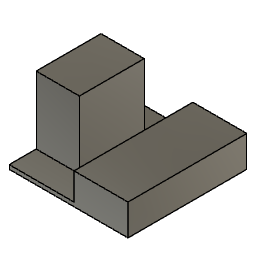
MotorDriver v2 (Autodesk Fusion 360 design; units mm, degrees)
Autodesk Fusion 360 part; units mm, degrees
sketch "Esquisse1" plane through (0, 0, 0) normal (0, 0, 1) x (1, 0, 0)
  line L0 (0, 0) -> (4.4, 0)
  line L1 (4.4, 0) -> (4.4, 4.4)
  line L2 (4.4, 4.4) -> (0, 4.4)
  line L3 (0, 4.4) -> (0, 0)
  dimension "d1" = 4.4
  dimension "d2" = 4.4
  constraint horizontal L0
  constraint vertical L1
  constraint horizontal L2
  constraint vertical L3
  constraint coincident L0.start L3.end
  measures "d1" distance of L0.start L0.end
  measures "d2" distance of L0.start L2.end
extrude "Extrusion1" add sketch "Esquisse1" along normal blind 0.15
sketch "Esquisse2" plane through (0, 0, 0.15) normal (0, 0, 1) x (-1, 0, 0)
  line L0 (0, -4.4) -> (0, 0)
  line L1 (0, 0) -> (-4.4, 0)
  line L2 (-4.4, 0) -> (-4.4, -4.4)
  line L3 (-4.4, -4.4) -> (0, -4.4)
  line L4 (-4.4, 0) -> (-2.4, 0)
  line L5 (-2.4, 0) -> (-2.4, -4.4)
  line L6 (-2.4, -4.4) -> (-4.4, -4.4)
  line L7 (-4.4, -4.4) -> (-4.4, 0)
  dimension "d5" = 2
  constraint horizontal L4
  constraint vertical L5
  constraint horizontal L6
  constraint vertical L7
  constraint coincident L3 L5.end
  constraint coincident L1.end L2.start
  measures "d5" distance of L1.end L4.end
extrude "Extrusion2" add sketch "Esquisse2" along normal blind 1 contours L1 L2 L3 L4 L5 L6 L7
sketch "Esquisse3" plane through (0, 0, 0.15) normal (0, 0, 1) x (-1, 0, 0)
  line L0 (-2.4, 0) -> (-2.4, -4.4)
  line L1 (-2.4, -4.4) -> (0, -4.4)
  line L2 (0, -4.4) -> (0, 0)
  line L3 (0, 0) -> (-2.4, 0)
  line L4 (0, -3.4) -> (-1.6, -3.4)
  line L5 (-1.6, -3.4) -> (-1.6, -1)
  line L6 (-1.6, -1) -> (0, -1)
  line L7 (0, -1) -> (0, -3.4)
  dimension "d8" = 1.6
  dimension "d9" = 2.4
  dimension "d11" = 1
  constraint horizontal L4
  constraint vertical L5
  constraint horizontal L6
  constraint vertical L7
  constraint coincident L2 L4.start
  measures "d8" distance of L4.start L4.end
  measures "d9" distance of L4.start L6.end
  measures "d11" distance of L3 L6
extrude "Extrusion3" add sketch "Esquisse3" along normal blind 2.5 contours L2 L4 L5 L6 L7
scale "Echelle1" factor 10 about (0, 3.4, 2.65) bodies 1
